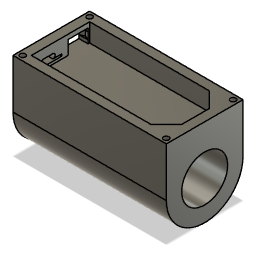
print_67f13b0424f398.35034424 (Autodesk Fusion 360 design; units mm, degrees)
Autodesk Fusion 360 part; units mm, degrees
note: some values were not read from the file. Set by a fixed rule: which sketch regions a step uses.
sketch "Sketch1" plane through (0, 0, 0) normal (1, 0, 0) x (0, 0, -1)
  line L0 (0, 0) -> (-50, 0)
  line L1 (-50, 0) -> (-50, 50)
  line L2 (-50, 50) -> (0, 50)
  line L3 (0, 50) -> (0, 0)
  constraint horizontal L0
  constraint vertical L1
  constraint horizontal L2
  constraint vertical L3
  constraint coincident L0.start L3.end
extrude "Extrude1" add sketch "Sketch1" along normal blind 100 makes body 1
ref_plane "WorkPlane1" through (50, 25, 25) normal (0, 1, 0) x (0, 0, 1)
sketch "Sketch2" plane through (0, 25, 0) normal (0, 1, 0) x (1, 0, 0)
  line L0 (0, -25) -> (0, -9.25)
  line L1 (10, -25) -> (10, -9.25)
  line L2 (20, -25) -> (20, -9.3)
  line L3 (30, -25) -> (30, -9.45)
  line L4 (40, -25) -> (40, -9.5)
  line L5 (50, -25) -> (50, -9.6)
  line L6 (60, -25) -> (60, -9.9)
  line L7 (70, -25) -> (70, -10)
  line L8 (80, -25) -> (80, -10)
  line L9 (90, -25) -> (90, -10)
  line L10 (100, -25) -> (100, -10)
  line L11 (0, -25) -> (100, -25)
  line L12 (0, -9.25) -> (10, -9.25)
  line L13 (10, -9.25) -> (20, -9.3)
  line L14 (20, -9.3) -> (30, -9.45)
  line L15 (30, -9.45) -> (40, -9.5)
  line L16 (40, -9.5) -> (50, -9.6)
  line L17 (50, -9.6) -> (60, -9.9)
  line L18 (60, -9.9) -> (70, -10)
  line L19 (70, -10) -> (80, -10)
  line L20 (80, -10) -> (90, -10)
  line L21 (100, -10) -> (90, -10)
  dimension "d4" = 15.75
  dimension "d5" = 15.75
  dimension "d6" = 15.7
  dimension "d7" = 15.55
  dimension "d8" = 15.5
  dimension "d9" = 15.4
  dimension "d10" = 15.1
  dimension "d11" = 15
  dimension "d12" = 15
  dimension "d13" = 15
  dimension "d14" = 15
  constraint vertical L0
  constraint vertical L1
  constraint vertical L2
  constraint vertical L3
  constraint vertical L4
  constraint vertical L5
  constraint parallel L5 L6
  constraint vertical L7
  constraint parallel L7 L8
  constraint parallel L8 L9
  constraint parallel L9 L10
  constraint perpendicular L10 L11
  constraint perpendicular L1 L12
  constraint perpendicular L8 L19
  constraint perpendicular L9 L20
  constraint perpendicular L9 L21
  measures "d4" distance of L0.start L0.end
  measures "d5" distance of L1.start L1.end
  measures "d6" distance of L2.start L2.end
  measures "d7" distance of L3.start L3.end
  measures "d8" distance of L4.start L4.end
  measures "d9" distance of L5.start L5.end
  measures "d10" distance of L6.start L6.end
  measures "d11" distance of L7.start L7.end
  measures "d12" distance of L8.start L8.end
  measures "d13" distance of L9.start L9.end
  measures "d14" distance of L10.start L10.end
revolve "Revolve1" cut sketch "Sketch2" angle 360 about axis through (0, 25, 25) along (1, 0, 0) bodies 1
sketch "Sketch15" plane through (100, 0, 0) normal (1, 0, 0) x (0, 0, -1)
  circle A0 centre (-25, 25) radius 15
  line L0 (0, 50) -> (-50, 50)
  line L1 (-50, 50) -> (-50, 0)
  line L2 (-50, 0) -> (0, 0)
  line L3 (0, 0) -> (0, 50)
fillet "Fillet1" radius 25 1 edges at (50, 0, 50) on bodies 1
fillet "Fillet2" radius 25 1 edges at (50, 0, 0) on bodies 1
sketch "Sketch17" plane through (0, 50, 0) normal (0, 1, 0) x (-1, 0, 0)
  line L0 (0, 0) -> (0, 50)
  line L1 (-100, 50) -> (-100, 0)
  line L2 (0, 50) -> (-100, 50)
  line L3 (-100, 0) -> (0, 0)
  line L4 (-94, 44) -> (-94, 6)
  line L5 (-94, 6) -> (-6, 6)
  line L6 (-6, 6) -> (-6, 44)
  line L7 (-6, 44) -> (-94, 44)
  dimension "d49" = -6
extrude "Extrude11" cut sketch "Sketch17" against normal blind 5 contours L4 L5 L6 L7 bodies 1
extrude "Extrude12" add 1 faces at (35.3333, 50, 48) along direction (0, 1, 0) blind 7 on bodies 1 bodies 1
sketch "Sketch18" plane through (0, 57, 0) normal (0, 1, 0) x (-1, 0, 0)
  line L0 (-94, 6) -> (-94, 44)
  line L1 (-94, 44) -> (-6, 44)
  line L2 (-6, 44) -> (-6, 6)
  line L3 (-6, 6) -> (-94, 6)
  line L4 (0, 0) -> (0, 50)
  line L5 (0, 50) -> (-100, 50)
  line L6 (-100, 50) -> (-100, 0)
  line L7 (-100, 0) -> (0, 0)
  circle A0 centre (-3.2, 3.2) radius 1.75
  circle A1 centre (-96.8, 3.2) radius 1.75
  circle A2 centre (-96.8, 46.8) radius 1.75
  circle A3 centre (-3.2, 46.8) radius 1.75
  dimension "d50" = 3.5
  dimension "d51" = 3.2
  dimension "d52" = 3.2
  dimension "d53" = 3.2
  dimension "d54" = 3.2
  constraint equal A0 A1
  constraint equal A1 A2
  constraint equal A2 A3
  constraint vertical A0.centre A3.centre
  constraint horizontal A0.centre A1.centre
  constraint vertical A1.centre A2.centre
  constraint horizontal A2.centre A3.centre
  measures "d50" diameter of A0
  measures "d51" distance of L7 A0.centre
  measures "d52" distance of L4 A0.centre
  measures "d53" distance of L6 A2.centre
  measures "d54" distance of L5 A2.centre
extrude "Extrude13" cut sketch "Sketch18" against normal blind 6 contours A0 | A1 | A2 | A3 bodies 1
sketch "Sketch19" plane through (0, 57, 0) normal (0, 1, 0) x (-1, 0, 0)
  circle A0 centre (-96.8, 3.2) radius 1.75
  circle A1 centre (-3.2, 46.8) radius 1.75
  circle A2 centre (-96.8, 46.8) radius 1.75
  circle A3 centre (-3.2, 3.2) radius 1.75
  line L0 (-94, 6) -> (-94, 44)
  line L1 (-94, 44) -> (-6, 44)
  line L2 (-6, 44) -> (-6, 6)
  line L3 (-6, 6) -> (-94, 6)
  line L4 (0, 0) -> (0, 50)
  line L5 (0, 50) -> (-100, 50)
  line L6 (-100, 50) -> (-100, 0)
  line L7 (-100, 0) -> (0, 0)
  line L8 (0, 0) -> (-100, 0)
  line L9 (-100, 0) -> (-100, 50)
  line L10 (-100, 50) -> (0, 50)
  line L11 (0, 50) -> (0, 0)
  circle A4 centre (-3.2, 3.2) radius 1.5
  circle A5 centre (-96.8, 3.2) radius 1.5
  circle A6 centre (-96.8, 46.8) radius 1.5
  circle A7 centre (-3.2, 46.8) radius 1.5
  dimension "d57" = 3
  dimension "d58" = 3
  dimension "d59" = 3
  dimension "d60" = 3
  constraint horizontal L8
  constraint vertical L9
  constraint horizontal L10
  constraint vertical L11
  constraint coincident L5.end L6.start
  constraint coincident L4.start L7.end
  constraint concentric A3 A4
  constraint concentric A0 A5
  constraint concentric A2 A6
  constraint concentric A1 A7
  measures "d57" diameter of A4
  measures "d58" diameter of A5
  measures "d59" diameter of A6
  measures "d60" diameter of A7
extrude "Extrude14" add sketch "Sketch19" along normal blind 3 from surface at 1 separate body contours L0 L1 L2 L3 | L4 L5 L6 L7 L8 L9 L10 L11 makes body 2
sketch "Sketch20" plane through (0, 61, 0) normal (0, 1, 0) x (-1, 0, 0)
  circle A0 centre (-3.2, 46.8) radius 1.75
  circle A1 centre (-3.2, 3.2) radius 1.75
  circle A2 centre (-96.8, 46.8) radius 1.75
  circle A3 centre (-96.8, 3.2) radius 1.75
  line L0 (0, 50) -> (-100, 50)
  line L1 (-100, 50) -> (-100, 0)
  line L2 (-100, 0) -> (0, 0)
  line L3 (0, 0) -> (0, 50)
  circle A4 centre (-3.2, 3.2) radius 2.75
  circle A5 centre (-96.8, 3.2) radius 2.75
  circle A6 centre (-96.8, 46.8) radius 2.75
  circle A7 centre (-3.2, 46.8) radius 2.75
  dimension "d64" = 5.5
  dimension "d65" = 5.5
  dimension "d66" = 5.5
  dimension "d67" = 5.5
  constraint concentric A1 A4
  constraint concentric A3 A5
  constraint concentric A2 A6
  constraint concentric A0 A7
  measures "d64" diameter of A4
  measures "d65" diameter of A5
  measures "d66" diameter of A6
  measures "d67" diameter of A7
extrude "Extrude15" cut sketch "Sketch20" against normal blind 1.5 contours A4 | A5 | A6 | A7 bodies 2
sketch "Sketch21" plane through (0, 45, 0) normal (0, 1, 0) x (-1, 0, 0)
  line L0 (-6, 44) -> (-94, 44)
  line L1 (-94, 44) -> (-94, 6)
  line L2 (-94, 6) -> (-6, 6)
  line L3 (-6, 6) -> (-6, 44)
sketch "Sketch22" plane through (0, 0, 0) normal (-1, 0, 0) x (0, 0, 1)
  circle A0 centre (25, 25) radius 15.75
  arc A1 (0, 25) -> (50, 25) centre (25, 25) ccw
  line L0 (50, 25) -> (50, 57)
  line L1 (50, 57) -> (0, 57)
  line L2 (0, 57) -> (0, 25)
  line L3 (7, 54) -> (20, 54)
  line L4 (20, 54) -> (20, 45)
  line L5 (20, 45) -> (7, 45)
  line L6 (7, 45) -> (7, 54)
  dimension "d72" = 13
  dimension "d73" = 9
  dimension "d74" = 7
  dimension "d75" = 3
  constraint horizontal L3
  constraint vertical L4
  constraint horizontal L5
  constraint vertical L6
  measures "d72" distance of L3.start L3.end
  measures "d73" distance of L3.end L4.end
  measures "d74" distance of L2 L6
  measures "d75" distance of L1 L3
extrude "Extrude16" cut sketch "Sketch22" against normal blind 6 contours L3 L4 L5 L6 bodies 1
sketch "Sketch25" plane through (0, 45, 0) normal (0, 1, 0) x (-1, 0, 0)
  line L0 (-6, 44) -> (-94, 44)
  line L1 (-94, 44) -> (-94, 6)
  line L2 (-94, 6) -> (-6, 6)
  line L3 (-6, 6) -> (-6, 7)
  line L4 (-6, 7) -> (0, 7)
  line L5 (0, 7) -> (0, 20)
  line L6 (0, 20) -> (-6, 20)
  line L7 (-6, 20) -> (-6, 44)
  line L8 (0, 7) -> (-3, 5.75)
  line L9 (-3, 5.75) -> (-6, 7)
  line L10 (0, 20) -> (-3, 21.25)
  line L11 (-3, 21.25) -> (-6, 20)
  line L12 (0, 20) -> (-6, 20)
  line L13 (0, 7) -> (-6, 7)
  dimension "d76" = 15.5
  constraint coincident L4.end L5.start
  constraint coincident L3.end L4.start
  constraint equal L8 L9
  constraint coincident L5.end L6.start
  constraint coincident L6.end L7.start
  constraint equal L10 L11
  constraint equal L9 L11
  measures "d76" distance of L8.end L10.end
extrude "Extrude17" cut sketch "Sketch25" along normal blind 4.5 from surface at 2.25 contours L6 L10 L11 L12 | L4 L8 L9 L13 bodies 1
sketch "Sketch26" plane through (0, 0, 0) normal (-1, 0, 0) x (0, 0, 1)
  line L0 (20, 54) -> (20, 51.75)
  line L1 (20, 51.75) -> (20, 47.25)
  line L2 (20, 47.25) -> (20, 45)
  line L3 (20, 45) -> (7, 45)
  line L4 (7, 45) -> (7, 47.25)
  line L5 (7, 47.25) -> (7, 51.75)
  line L6 (7, 51.75) -> (7, 54)
  line L7 (7, 54) -> (20, 54)
  circle A0 centre (25, 25) radius 15.75
  arc A1 (0, 25) -> (50, 25) centre (25, 25) ccw
  line L8 (50, 25) -> (50, 57)
  line L9 (50, 57) -> (0, 57)
  line L10 (0, 57) -> (0, 25)
  line L11 (30, 51) -> (36, 51)
  line L12 (30, 48) -> (36, 48)
  line L13 (20, 54) -> (20, 49.5) construction
  line L14 (20, 49.5) -> (20, 45) construction
  arc A2 (30, 51) -> (30, 48) centre (30, 49.5) ccw
  arc A3 (36, 48) -> (36, 51) centre (36, 49.5) ccw
  dimension "d80" = 3
  dimension "d81" = 9
  dimension "d83" = 14
  constraint equal A2 A3
  constraint horizontal A2.centre A3.centre
  constraint tangent L11 A3
  constraint tangent L12 A3
  constraint horizontal L11
  constraint horizontal L12
  constraint coincident L0.start L7.end
  constraint coincident L1 L13.end
  constraint perpendicular L7 L13
  constraint coincident L2.end L3.start
  constraint perpendicular L3 L14
  constraint equal L13 L14
  constraint horizontal A2.centre L13.end
  measures "d80" diameter of A2
  measures "d83" distance of L8 A3.centre
extrude "Extrude18" cut sketch "Sketch26" against normal up to surface (6 mm away) contours L11 L12 A2 A3 bodies 1
sketch "Sketch27" plane through (6, 0, 0) normal (1, 0, 0) x (0, 0, -1)
  line L0 (-36, 51) -> (-30, 51)
  arc A0 (-30, 48) -> (-30, 51) centre (-30, 49.5) ccw
  line L1 (-30, 48) -> (-36, 48)
  arc A1 (-36, 51) -> (-36, 48) centre (-36, 49.5) ccw
  line L2 (-7, 54) -> (-7, 51.75)
  line L3 (-7, 51.75) -> (-7, 47.25)
  line L4 (-7, 47.25) -> (-7, 45)
  line L5 (-7, 45) -> (-6, 45)
  line L6 (-6, 45) -> (-6, 57)
  line L7 (-6, 57) -> (-44, 57)
  line L8 (-44, 57) -> (-44, 45)
  line L9 (-44, 45) -> (-20, 45)
  line L10 (-20, 45) -> (-20, 47.25)
  line L11 (-20, 47.25) -> (-20, 51.75)
  line L12 (-20, 51.75) -> (-20, 54)
  line L13 (-20, 54) -> (-7, 54)
  line L14 (-30, 51) -> (-36, 51)
  arc A2 (-36, 51) -> (-36, 48) centre (-36, 49.5) ccw
  line L15 (-30, 48) -> (-36, 48)
  arc A3 (-30, 48) -> (-30, 51) centre (-30, 49.5) ccw
  line L16 (-41.8, 46.7) -> (-24.2, 46.7)
  line L17 (-24.2, 46.7) -> (-24.2, 48)
  line L18 (-24.2, 48) -> (-41.8, 48)
  line L19 (-41.8, 48) -> (-41.8, 46.7)
  line L20 (-33, 51) -> (-33, 48) construction
  dimension "d86" = 17.6
  dimension "d87" = 1.3
  constraint horizontal L16
  constraint vertical L17
  constraint horizontal L18
  constraint vertical L19
  constraint collinear L1 L18
  constraint midpoint L14 L20.start
  constraint midpoint L15 L20.end
  measures "d86" distance of L17 L19
  measures "d87" distance of L16 L18
extrude "Extrude19" cut sketch "Sketch27" against normal up to surface (4.5 mm away) contours L1 L15 L16 L17 L18 L19 bodies 1
chamfer "Chamfer1" distance 10 angle 45 2 edges at (94, 51, 6) (94, 51, 44) on bodies 1
hidden bodies 2
equation "d52 = d51"
equation "d53 = d51"
equation "d54 = d51"
equation "d58 = d57"
equation "d59 = d57"
equation "d60 = d57"
equation "d65 = d64"
equation "d66 = d64"
equation "d67 = d64"
